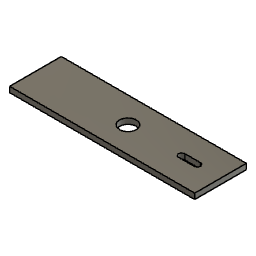
AE361 v4 (Autodesk Fusion 360 design; units mm, degrees)
Autodesk Fusion 360 part; units mm, degrees
sketch "Sketch1" plane through (0, 0, 0) normal (0, 1, 0) x (1, 0, 0)
  line L0 (0, 0) -> (-118.2, 0)
  line L1 (-118.2, 0) -> (-118.2, 32.98)
  line L2 (-118.2, 32.98) -> (0, 32.98)
  line L3 (0, 32.98) -> (0, 0)
  line L4 (0, 0) -> (0, 16.49)
  line L5 (-118.2, 16.49) -> (0, 16.49)
  circle A0 centre (-59.1, 16.49) radius 5.37
  point P0 (-59.1, 16.49)
  dimension "d1" = 118.2
  dimension "d2" = 32.98
  dimension "d3" = 10.74
  dimension "d4" = 59.1
  constraint horizontal L0
  constraint vertical L1
  constraint horizontal L2
  constraint vertical L3
  constraint coincident L0.start L3.end
  constraint midpoint L3 L4.end
  constraint midpoint L1 L5.start
  constraint midpoint L5 P0
  constraint coincident P0 A0.centre
  measures "d1" distance of L0.start L0.end
  measures "d2" distance of L0.start L2.end
  measures "d3" diameter of A0
  measures "d4" distance of L4.end P0
sketch "Sketch2" plane through (0, 0, 0) normal (0, 1, 0) x (1, 0, 0)
  line L0 (-15.0272, 18.6866) -> (-25, 18.6866)
  arc A0 (-25, 18.6866) -> (-25, 14.6866) centre (-25, 16.6866) ccw
  line L1 (-25, 14.6866) -> (-15.0272, 14.6866)
  arc A1 (-15.0272, 14.6866) -> (-15.0272, 18.6866) centre (-15.0272, 16.6866) ccw
  line L2 (-15.0272, 16.6866) -> (-25, 16.6866) construction
  dimension "d5" = 4
  constraint tangent L0 A0
  constraint tangent A0 L1
  constraint parallel L0 L1
  constraint tangent L1 A1
  constraint tangent L0 A1
  constraint horizontal L2
  measures "d5" diameter of A0
extrude "Extrude1" add sketch "Sketch1" against normal blind 4 contours L0 L1 L3 L4 L5 A0 | L1 L2 L3 L5 A0
extrude "Extrude2" cut sketch "Sketch2" against normal blind 4
move_face "OffsetFaces1" offset -0.5 1 faces at (-100.29, 0, -16.49)
sketch "Sketch3" plane through (0, 0, 0) normal (0, 1, 0) x (1, 0, 0)
sketch "Sketch4" plane through (0, 0, 0) normal (0, 1, 0) x (1, 0, 0)
